cnc circuit box (Autodesk Fusion 360 design; units mm, degrees)
Autodesk Fusion 360 part; units mm, degrees
note: some values were not read from the file. Set by a fixed rule: which sketch regions a step uses.
sketch "Sketch1" plane through (0, 0, 0) normal (0, 1, 0) x (1, 0, 0)
  line L0 (0, 0) -> (90, 0)
  line L1 (90, 0) -> (90, -52)
  line L2 (90, -52) -> (0, -52)
  line L3 (0, -52) -> (0, 0)
  line L4 (2.5, -2.5) -> (87.5, -2.5)
  line L5 (87.5, -2.5) -> (87.5, -49.5)
  line L6 (87.5, -49.5) -> (2.5, -49.5)
  line L7 (2.5, -49.5) -> (2.5, -2.5)
  line L8 (0, 0) -> (90, 0)
  line L9 (90, 0) -> (90, -8)
  line L10 (90, -8) -> (0, -8)
  line L11 (0, -8) -> (0, 0)
  circle A0 centre (2.5, -2.5) radius 1
  circle A1 centre (87.5, -2.5) radius 1
  circle A2 centre (2.5, -49.5) radius 1
  circle A3 centre (87.5, -49.5) radius 1
  line L12 (91.5, -53.5) -> (-1.5, -53.5)
  line L13 (-1.5, -53.5) -> (-1.5, 1.5)
  line L14 (-1.5, 1.5) -> (91.5, 1.5)
  line L15 (91.5, 1.5) -> (91.5, -53.5)
  line L16 (-3.5, 3.5) -> (93.5, 3.5)
  line L17 (93.5, 3.5) -> (93.5, -55.5)
  line L18 (93.5, -55.5) -> (-3.5, -55.5)
  line L19 (-3.5, -55.5) -> (-3.5, 3.5)
  line L20 (45, -8) -> (80, -8)
  line L21 (80, -8) -> (80, 3.5)
  line L22 (80, 3.5) -> (45, 3.5)
  line L23 (45, 3.5) -> (45, -8)
  line L24 (45, -8) -> (10, -8)
  line L25 (10, -8) -> (10, 3.5)
  line L26 (10, 3.5) -> (45, 3.5)
  line L27 (45, 3.5) -> (45, -8)
  line L28 (10, 3.5) -> (80, 3.5)
  line L29 (80, 3.5) -> (80, -8)
  line L30 (80, -8) -> (10, -8)
  line L31 (10, -8) -> (10, 3.5)
  dimension "d1" = 90
  dimension "d2" = 52
  dimension "d3" = 2.5
  dimension "d4" = 8
  dimension "d5" = 2
  dimension "d6" = 2
  dimension "d7" = 2
  dimension "d8" = 2
  dimension "d13" = 1.5
  dimension "d14" = 3.5
  dimension "d44" = 35
  dimension "d45" = 35
  constraint horizontal L0
  constraint vertical L1
  constraint horizontal L2
  constraint vertical L3
  constraint coincident L0.start L3.end
  constraint horizontal L8
  constraint vertical L9
  constraint horizontal L10
  constraint vertical L11
  constraint coincident L4.start L7.end
  constraint coincident L4.end L5.start
  constraint coincident L6.end L7.start
  constraint coincident L5.end L6.start
  constraint horizontal L20
  constraint vertical L21
  constraint horizontal L22
  constraint vertical L23
  constraint midpoint L10 L20.start
  constraint horizontal L24
  constraint vertical L25
  constraint horizontal L26
  constraint vertical L27
  constraint horizontal L28
  constraint vertical L29
  constraint horizontal L30
  constraint vertical L31
  measures "d1" distance of L0.start L0.end
  measures "d2" distance of L0.start L2.end
  measures "d4" distance of L0.start L10.end
  measures "d5" diameter of A0
  measures "d6" diameter of A1
  measures "d7" diameter of A2
  measures "d8" diameter of A3
  measures "d44" distance of L20.start L20.end
  measures "d45" distance of L20.start L24.end
extrude "Extrude1" add sketch "Sketch1" against normal blind 10 contours L0 L3 L4 L7 L8 L10 L11 A0 L25 L31 | L0 L4 L8 L23 L25 L27 L31 | L1 L2 L3 L5 L6 L7 L10 A2 A3 | L0 L4 L8 L21 L23 L27 L29 | L4 L7 L10 A0 L25 L31 | L4 L10 L23 L24 L25 L27 L30 L31 | L5 L6 L7 L10 A2 A3 L20 L24 L30 | L0 L1 L4 L5 L8 L9 L10 A1 L21 L29 | L4 L10 L20 L21 L23 L27 L29 L30 | L4 L7 A0 | L4 L7 A0 | L6 L7 A2 | L6 L7 A2 | L4 L5 L10 A1 L21 L29 | L4 L5 A1 | L4 L5 A1 | L5 L6 A3 | L5 L6 A3
extrude "Extrude2" add sketch "Sketch1" along normal blind 10 contours L4 L7 A0 | L4 L7 A0 | L6 L7 A2 | L6 L7 A2 | L4 L5 A1 | L4 L5 A1 | L5 L6 A3 | L5 L6 A3
sketch "Sketch2" plane through (0, -10, 0) normal (0, -1, 0) x (1, 0, 0)
  line L0 (0, 52) -> (0, 0)
  line L1 (0, 0) -> (90, 0)
  line L2 (90, 0) -> (90, 52)
  line L3 (90, 52) -> (0, 52)
  line L4 (0, 52) -> (0, 0)
  circle A0 centre (84, 38.5) radius 2.5
  circle A1 centre (84, 13.4738) radius 2.5
  circle A2 centre (6, 38.5) radius 2.5
  circle A3 centre (6, 13.5) radius 2.5
  circle A4 centre (6, 38.5) radius 4.5
  circle A5 centre (6, 13.5) radius 4.5
  circle A6 centre (84, 13.4738) radius 4.5
  circle A7 centre (84, 38.5) radius 4.5
  circle A8 centre (6, 38.5) radius 5.5
  circle A9 centre (6, 13.5) radius 5.5
  circle A10 centre (84, 13.4738) radius 5.5
  circle A11 centre (84, 38.5) radius 5.5
  dimension "d19" = 5
  dimension "d21" = 5
  dimension "d22" = 5
  dimension "d23" = 9
  dimension "d24" = 9
  dimension "d25" = 9
  dimension "d26" = 9
  dimension "d27" = 11
  dimension "d28" = 11
  dimension "d29" = 11
  dimension "d30" = 11
  constraint coincident L0.start L3.end
  constraint coincident L0.end L1.start
  constraint concentric A2 A4
  constraint concentric A3 A5
  constraint concentric A1 A6
  constraint concentric A0 A7
  constraint concentric A4 A8
  constraint concentric A5 A9
  constraint concentric A6 A10
  constraint concentric A7 A11
  measures "d19" diameter of A0
  measures "d21" diameter of A2
  measures "d22" diameter of A3
  measures "d23" diameter of A4
  measures "d24" diameter of A5
  measures "d25" diameter of A6
  measures "d26" diameter of A7
  measures "d27" diameter of A8
  measures "d28" diameter of A9
  measures "d29" diameter of A10
  measures "d30" diameter of A11
extrude "Extrude3" cut sketch "Sketch2" against normal blind 1 contours L0 L1 L2 L3 L4
extrude "Extrude4" cut sketch "Sketch2" against normal blind 20 contours A0 | A1 | A2 | A3
extrude "Extrude5" add sketch "Sketch1" against normal blind 2 contours L0 L1 L2 L3 L8 L9 L11 L12 L13 L14 L15 L21 L25 L29 L31 | L0 L8 L14 L23 L25 L27 L31 | L0 L8 L14 L21 L23 L27 L29 | L14 L16 L23 L25 L26 L27 L28 L31 | L12 L13 L14 L15 L16 L17 L18 L19 L21 L25 L29 L31 | L14 L16 L21 L22 L23 L27 L28 L29
extrude "Extrude6" add sketch "Sketch1" along normal blind 25 contours L14 L16 L23 L25 L26 L27 L28 L31 | L12 L13 L14 L15 L16 L17 L18 L19 L21 L25 L29 L31 | L14 L16 L21 L22 L23 L27 L28 L29
extrude "Extrude7" cut 4 faces at (2.7626, 10, 49.9696) (87.8185, 10, 48.9483) (87.2491, 10, 3.0466) (2.3333, 10, 2.7887) along direction (0, -1, 0) blind 7
extrude "Extrude8" cut 4 faces at (88.4795, -10, 13.2006) (88.4795, -10, 38.2268) (10.4795, -10, 13.2268) (10.4795, -10, 38.2268) along direction (0, 1, 0) blind 5
extrude "Extrude9" cut sketch "Sketch1" along normal blind 28 contours L0 L8 L14 L23 L25 L27 L31 | L0 L4 L8 L23 L25 L27 L31 | L0 L8 L14 L21 L23 L27 L29 | L0 L4 L8 L21 L23 L27 L29 | L4 L10 L23 L24 L25 L27 L30 L31 | L14 L16 L23 L25 L26 L27 L28 L31 | L14 L16 L21 L22 L23 L27 L28 L29 | L4 L10 L20 L21 L23 L27 L29 L30
sketch "Sketch3" plane through (91.5, 0, 0) normal (-1, 0, 0) x (0, 0, 1)
  line L0 (-1.5, 0) -> (53.5, 0)
  line L1 (53.5, 0) -> (53.5, 25)
  line L2 (53.5, 25) -> (-1.5, 25)
  line L3 (-1.5, 25) -> (-1.5, 0)
  line L4 (26, 25) -> (26, 23)
  line L5 (26, 23) -> (31, 23)
  line L6 (31, 23) -> (31, 22)
  line L7 (31, 22) -> (26, 22)
  line L8 (26, 22) -> (26, 23)
  line L9 (31, 23) -> (21, 23)
  line L10 (21, 23) -> (21, 22)
  line L11 (21, 22) -> (31, 22)
  line L12 (31, 22) -> (31, 23)
  dimension "d48" = 2
  constraint midpoint L2 L4.start
  constraint horizontal L5
  constraint vertical L6
  constraint horizontal L7
  constraint vertical L8
  constraint horizontal L9
  constraint vertical L10
  constraint horizontal L11
  constraint vertical L12
  measures "d48" distance of L4.start L4.end
extrude "Extrude10" cut sketch "Sketch3" against normal blind 1 contours L5 L6 L7 L8 L9 L11 L12 | L8 L9 L10 L11
sketch "Sketch4" plane through (-1.5, 0, 0) normal (1, 0, 0) x (0, 0, -1)
  line L0 (-53.5, 0) -> (1.5, 0)
  line L1 (1.5, 0) -> (1.5, 25)
  line L2 (1.5, 25) -> (-53.5, 25)
  line L3 (-53.5, 25) -> (-53.5, 0)
  line L4 (-53.5, 25) -> (1.5, 25)
  line L5 (-26, 25) -> (-21, 25)
  line L6 (-21, 25) -> (-21, 23)
  line L7 (-21, 23) -> (-31, 23)
  line L8 (-31, 23) -> (-31, 22)
  line L9 (-31, 22) -> (-21, 22)
  line L10 (-21, 22) -> (-21, 23)
  dimension "d51" = 5
  dimension "d52" = 10
  dimension "d53" = 1
  constraint coincident L2.end L3.start
  constraint coincident L1.end L2.start
  constraint midpoint L4 L5.start
  constraint perpendicular L2 L6
  constraint horizontal L7
  constraint vertical L8
  constraint horizontal L9
  constraint vertical L10
  measures "d51" distance of L5.start L5.end
  measures "d52" distance of L6.end L7.end
  measures "d53" distance of L6.end L9.end
extrude "Extrude11" cut sketch "Sketch4" against normal blind 1 contours L7 L8 L9 L10
sketch "Sketch5" plane through (0, 0, 0) normal (0, 1, 0) x (1, 0, 0)
  line L0 (0, -52) -> (0, -48)
  line L1 (0, -48) -> (0, -23)
  line L2 (0, -52) -> (0, -33)
  line L3 (0, -48) -> (0, -23)
  line L4 (0, -23) -> (-9, -23)
  line L5 (-1.5, 1.5) -> (-1.5, -53.5)
  line L6 (-9, -48) -> (-1.5, -48)
  line L7 (-9, -48) -> (-9, -23)
  line L8 (-1.5, -48) -> (-1.5, -33)
  line L9 (-1.5, -33) -> (-3.5, -33)
  line L10 (-3.5, -33) -> (-3.5, -48)
  line L11 (-3.5, -48) -> (-1.5, -48)
  line L12 (-1.5, -48) -> (-1.5, -33)
  line L13 (-1.5, -23) -> (-3.5, -23)
  line L14 (-3.5, -23) -> (-3.5, -33)
  line L15 (-3.5, -33) -> (-1.5, -33)
  line L16 (-1.5, -33) -> (-1.5, -23)
  point P0 (0, -52)
  dimension "d56" = 4
  dimension "d57" = 25
  dimension "d58" = 19
  dimension "d59" = 15
  constraint coincident P0 L0.start
  constraint parallel L1 L3
  constraint perpendicular L1 L4
  constraint coincident L5 L6.end
  constraint perpendicular L1 L6
  constraint perpendicular L4 L7
  constraint horizontal L9
  constraint vertical L10
  constraint horizontal L11
  constraint vertical L12
  constraint coincident L6 L10.end
  constraint horizontal L13
  constraint vertical L14
  constraint horizontal L15
  constraint vertical L16
  constraint coincident L4 L13.start
  constraint coincident L5 L13.start
  measures "d56" distance of P0 L0.end
  measures "d57" distance of L0.end L1.end
  measures "d58" distance of P0 L2.end
  measures "d59" distance of L6.end L8.end
extrude "Extrude13" cut sketch "Sketch5" along normal blind 15 contours L4 L5 L9 L13 L14 L15 L16
extrude "Extrude12" cut sketch "Sketch5" along normal blind 8 contours L5 L6 L8 L9 L10 L11 L12 L15
extrude "Extrude14" add 1 faces at (30, -2, -2.3333) along direction (0, -1, 0) blind 7
extrude "Extrude15" add 4 faces at (88.4795, -5, 38.2268) (10.4795, -5, 38.2268) (10.4795, -5, 13.2268) (88.4795, -5, 13.2006) along direction (0, -1, 0) blind 4
sketch "Sketch6" plane through (0, 0, 0) normal (0, 1, 0) x (-1, 0, 0)
  line L0 (-10, -1.5) -> (1.5, -1.5)
  line L1 (1.5, -1.5) -> (1.5, 23)
  line L2 (1.5, 23) -> (3.5, 23)
  line L3 (3.5, 23) -> (3.5, 48)
  line L4 (3.5, 48) -> (1.5, 48)
  line L5 (1.5, 48) -> (1.5, 53.5)
  line L6 (1.5, 53.5) -> (-91.5, 53.5)
  line L7 (-91.5, 53.5) -> (-91.5, -1.5)
  line L8 (-91.5, -1.5) -> (-80, -1.5)
  line L9 (-80, -1.5) -> (-80, -3.5)
  line L10 (-80, -3.5) -> (-10, -3.5)
  line L11 (-10, -3.5) -> (-10, -1.5)
  circle A0 centre (-6, 13.5) radius 2.5
  circle A1 centre (-84, 13.4738) radius 2.5
  circle A2 centre (-6, 38.5) radius 2.5
  circle A3 centre (-84, 38.5) radius 2.5
  circle A4 centre (-2.5, 2.5) radius 1
  circle A5 centre (-87.5, 2.5) radius 1
  circle A6 centre (-2.5, 49.5) radius 1
  circle A7 centre (-87.5, 49.5) radius 1
  circle A8 centre (-6, 13.5) radius 4.5
  circle A9 centre (-84, 13.4738) radius 4.5
  circle A10 centre (-6, 38.5) radius 4.5
  circle A11 centre (-84, 38.5) radius 4.5
  dimension "d68" = 9
  dimension "d69" = 9
  dimension "d70" = 9
  dimension "d71" = 9
  constraint concentric A0 A8
  constraint concentric A1 A9
  constraint concentric A2 A10
  constraint concentric A3 A11
  measures "d68" diameter of A8
  measures "d69" diameter of A9
  measures "d70" diameter of A10
  measures "d71" diameter of A11
extrude "Extrude16" cut sketch "Sketch6" against normal blind 6 contours A8 | A9 | A10 | A11
sketch "Sketch7" plane through (0, 0, 0) normal (0, 1, 0) x (-1, 0, 0)
  circle A0 centre (-6, 38.5) radius 4.5
  circle A1 centre (-84, 38.5) radius 4.5
  circle A2 centre (-6, 13.5) radius 4.5
  circle A3 centre (-84, 13.4738) radius 4.5
  line L0 (-10, -1.5) -> (1.5, -1.5)
  line L1 (1.5, -1.5) -> (1.5, 23)
  line L2 (1.5, 23) -> (3.5, 23)
  line L3 (3.5, 23) -> (3.5, 48)
  line L4 (3.5, 48) -> (1.5, 48)
  line L5 (1.5, 48) -> (1.5, 53.5)
  line L6 (1.5, 53.5) -> (-91.5, 53.5)
  line L7 (-91.5, 53.5) -> (-91.5, -1.5)
  line L8 (-91.5, -1.5) -> (-80, -1.5)
  line L9 (-80, -1.5) -> (-80, -3.5)
  line L10 (-80, -3.5) -> (-10, -3.5)
  line L11 (-10, -3.5) -> (-10, -1.5)
  circle A4 centre (-2.5, 2.5) radius 1
  circle A5 centre (-87.5, 2.5) radius 1
  circle A6 centre (-2.5, 49.5) radius 1
  circle A7 centre (-87.5, 49.5) radius 1
  line L12 (-6, 13.5) -> (-84, 13.5)
  line L13 (-84, 13.5) -> (-84, 38.5)
  line L14 (-84, 38.5) -> (-6, 38.5)
  line L15 (-6, 38.5) -> (-6, 13.5)
  line L16 (-6, 38.5) -> (-84, 38.5)
  line L17 (-84, 38.5) -> (-84, 46.5)
  line L18 (-84, 46.5) -> (-6, 46.5)
  line L19 (-6, 46.5) -> (-6, 38.5)
  line L20 (-6, 13.5) -> (-84, 13.5)
  line L21 (-84, 13.5) -> (-84, 5.5)
  line L22 (-84, 5.5) -> (-6, 5.5)
  line L23 (-6, 5.5) -> (-6, 13.5)
  line L24 (-6, 5.5) -> (-14, 5.5)
  line L25 (-14, 5.5) -> (-14, 46.5)
  line L26 (-14, 46.5) -> (-6, 46.5)
  line L27 (-6, 46.5) -> (-6, 5.5)
  line L28 (-84, 5.5) -> (-76, 5.5)
  line L29 (-76, 5.5) -> (-76, 46.5)
  line L30 (-76, 46.5) -> (-84, 46.5)
  line L31 (-84, 46.5) -> (-84, 5.5)
  dimension "d74" = 8
  dimension "d75" = 8
  dimension "d76" = 8
  dimension "d77" = 8
  constraint horizontal L12
  constraint vertical L13
  constraint horizontal L14
  constraint vertical L15
  constraint coincident A1.centre L13.end
  constraint coincident A2.centre L12.start
  constraint horizontal L16
  constraint vertical L17
  constraint horizontal L18
  constraint vertical L19
  constraint horizontal L20
  constraint vertical L21
  constraint horizontal L22
  constraint vertical L23
  constraint horizontal L24
  constraint vertical L25
  constraint horizontal L26
  constraint vertical L27
  constraint horizontal L28
  constraint vertical L29
  constraint horizontal L30
  constraint vertical L31
  measures "d74" distance of A0.centre L18.end
  measures "d75" distance of A2.centre L22.end
  measures "d76" distance of L22.end L24.end
  measures "d77" distance of L21.end L28.end
extrude "Extrude17" cut sketch "Sketch7" against normal blind 8 contours L12 L14 L16 L20 L25 L29
fillet "Fillet2" radius 8 4 edges at (45, 0, 38.5) (76, 0, 26) (45, 0, 13.5) (14, 0, 26)
sketch "Sketch8" plane through (0, 0, 0) normal (0, 1, 0) x (-1, 0, 0)
  circle A0 centre (-87.5, 49.5) radius 1
  circle A1 centre (-2.5, 49.5) radius 1
  circle A2 centre (-87.5, 2.5) radius 1
  circle A3 centre (-2.5, 2.5) radius 1
  line L0 (-10, -1.5) -> (1.5, -1.5)
  line L1 (1.5, -1.5) -> (1.5, 23)
  line L2 (1.5, 23) -> (3.5, 23)
  line L3 (3.5, 23) -> (3.5, 48)
  line L4 (3.5, 48) -> (1.5, 48)
  line L5 (1.5, 48) -> (1.5, 53.5)
  line L6 (1.5, 53.5) -> (-91.5, 53.5)
  line L7 (-91.5, 53.5) -> (-91.5, -1.5)
  line L8 (-91.5, -1.5) -> (-80, -1.5)
  line L9 (-80, -1.5) -> (-80, -3.5)
  line L10 (-80, -3.5) -> (-10, -3.5)
  line L11 (-10, -3.5) -> (-10, -1.5)
  line L12 (-6, 34) -> (-6, 18)
  arc A4 (-6, 9) -> (-6, 18) centre (-6, 13.5) ccw
  line L13 (-6, 9) -> (-6, 5.5)
  line L14 (-6, 5.5) -> (-84, 5.5)
  line L15 (-84, 5.5) -> (-84, 8.9738)
  arc A5 (-84, 17.9738) -> (-84, 8.9738) centre (-84, 13.4738) ccw
  line L16 (-84, 17.9738) -> (-84, 34)
  arc A6 (-84, 43) -> (-84, 34) centre (-84, 38.5) ccw
  line L17 (-84, 43) -> (-84, 46.5)
  line L18 (-84, 46.5) -> (-6, 46.5)
  line L19 (-6, 46.5) -> (-6, 43)
  arc A7 (-6, 34) -> (-6, 43) centre (-6, 38.5) ccw
sketch "Sketch9" plane through (0, 0, 0) normal (0, 1, 0) x (-1, 0, 0)
sketch "Sketch10" plane through (0, 0, 0) normal (0, 1, 0) x (-1, 0, 0)
  line L0 (3.5, 48) -> (1.5, 48)
  line L1 (1.5, 48) -> (1.5, 23)
  line L2 (1.5, 23) -> (3.5, 23)
  line L3 (3.5, 23) -> (3.5, 48)
  line L4 (1.5, 53.5) -> (1.5, -1.5)
  constraint horizontal L0
  constraint vertical L1
  constraint horizontal L2
  constraint vertical L3
  constraint coincident L1.end L4
extrude "Extrude18" add sketch "Sketch10" along normal blind 2
extrude "Extrude19" cut 1 faces at (-2.1667, 8, 43) along direction (0, 1, 0) blind 4
extrude "Extrude20" cut 1 faces at (-2.8333, 15, 26.3333) along direction (0, 1, 0) blind 4
extrude "Extrude21" add 1 faces at (-3.5, 6, 5.3333) along direction (-1, 0, 0) blind 2
extrude "Extrude22" add 1 faces at (-0.3333, 5.3333, -3.5) along direction (0, 0, -1) blind 2
extrude "Extrude23" add 1 faces at (60.5, 2.3333, 55.5) along direction (0, 0, 1) blind 2
extrude "Extrude24" add 1 faces at (93.5, 2.3333, 36.5) along direction (1, 0, 0) blind 2
extrude "Extrude25" add 4 faces at (87.8185, 3, 48.9483) (2.7626, 3, 49.9696) (2.3333, 3, 2.7887) (87.2491, 3, 3.0466) along direction (0, 1, 0) blind 4
extrude "Extrude26" add 1 faces at (29.5, 25, 56.1667) along direction (0, 1, 0) blind 5
equation "d14 = 1.5 mm + 2 mm"
